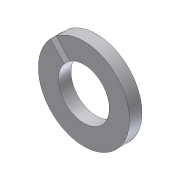
# Autodesk Inventor part: HW-00064
Saved by Autodesk Inventor 2012 (Build 160160000, 160)
## iProperties
Created: 2011-10-18
Part Number: HW-00064
Description: Washer, Lock 3/8"
Document SubType Name: Modeling
Designer: dfoster
Density: 1 g/cm^3
Mass: 0.369839 g
Surface Area: 5.23037 cm^2
Volume: 0.369839 cm^3
Material: Default
Title: Washer, Lock 3/8"
Author: dfoster
Autodesk Inventor part; units mm, degrees
ref_plane "YZ Plane" through (0, 0, 0) normal (1, 0, 0) x (0, 1, 0)
ref_plane "XZ Plane" through (0, 0, 0) normal (0, 1, 0) x (-1, 0, 0)
ref_plane "XY Plane" through (0, 0, 0) normal (0, 0, 1) x (1, 0, 0)
sketch "Sketch1" plane through (0, 0, 0) normal (0, 0, 1) x (1, 0, 0)
  arc A0 (-6.356, 5.8465) -> (-5.2294, 6.8727) centre (0, 0) ccw
  arc A1 (-3.7723, 3.0099) -> (-2.6457, 4.0362) centre (0, 0) ccw
  line L0 (-3.7723, 3.0099) -> (-6.356, 5.8465)
  line L1 (-5.2294, 6.8727) -> (-2.6457, 4.0362)
  line L2 (-6.9725, 7.6548) -> (-2.002, 2.1979)
  dimension "d0" = 17.272
  dimension "d1" = 9.652
  dimension "d2" = 1.524
  dimension "d3" = 0.762
  constraints: 6 end point, 4 point on circle, 2 centre point, 2 coincident, 2 parallel, 1 point on line
  measures "d0" diameter of A0
  measures "d1" diameter of A1
  measures "d2" distance between parallel lines of L1 L0
  measures "d3" distance between parallel lines of L2 L0
extrude "Extrusion1" add sketch "Sketch1" along normal blind 2.3813
equation "\"d3\" = 0.5 * d2"
body "Solid1"
